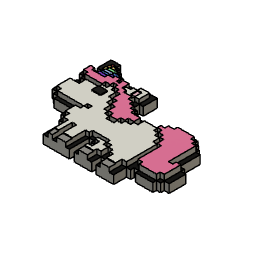
unicorn (Autodesk Fusion 360 design; units mm, degrees)
Autodesk Fusion 360 part; units mm, degrees
note: some values were not read from the file. Chosen so that the rebuilt part matches the saved one: which face or edge a step refers to; which pieces of a blend or face edit are solid.
sketch "Sketch2" plane through (0, 0, 0) normal (0, 0, 1) x (1, 0, 0)
  line L0 (0.8513, 43.4126) -> (0.8513, 31.4048)
  line L1 (0.8513, 31.4048) -> (4, 31.4048)
  line L2 (4, 31.4048) -> (4, 29)
  line L3 (4, 29) -> (7.2062, 29)
  line L4 (7.2062, 29) -> (7.2062, 31.4048)
  line L5 (7.2062, 31.4048) -> (4, 31.4048)
  line L6 (4, 41) -> (4, 31.4048)
  line L7 (4, 41) -> (10.3467, 41)
  line L8 (10.3467, 41) -> (10.3467, 46)
  line L9 (10.3467, 46) -> (19.3248, 46)
  line L10 (19.3248, 46) -> (19.3248, 48.3635)
  line L11 (19.3248, 48.3635) -> (7, 48.3635)
  line L12 (7, 48.3635) -> (7, 46)
  line L13 (7, 46) -> (4, 46)
  line L14 (4, 46) -> (4, 43.4126)
  line L15 (4, 43.4126) -> (0.8513, 43.4126)
  line L16 (1, 58) -> (1, 50.5063)
  line L17 (1, 50.5063) -> (4, 50.5063)
  line L18 (4, 50.5063) -> (4, 55.5959)
  line L19 (4, 55.5959) -> (7, 55.5959)
  line L20 (7, 55.5959) -> (7, 53.5)
  line L21 (7, 53.5) -> (10, 53.5)
  line L22 (10, 53.5) -> (10, 60.5)
  line L23 (10, 60.5) -> (7.5, 60.5)
  line L24 (7.5, 60.5) -> (7.5, 58)
  line L25 (7.5, 58) -> (1, 58)
  line L26 (4, 50.5063) -> (4, 48.3635)
  line L27 (4, 48.3635) -> (7, 48.3635)
  line L28 (7, 50.5063) -> (4, 50.5063)
  line L29 (7, 50.5063) -> (7, 48.3635)
  line L30 (7.5, 60.5) -> (7.5, 67.5)
  line L31 (7.5, 67.5) -> (10.5, 67.5)
  line L32 (10.5, 67.5) -> (10.5, 70.311)
  line L33 (10.5, 70.311) -> (3.9179, 70.311)
  line L34 (3.9179, 70.311) -> (3.9179, 60.5)
  line L35 (3.9179, 60.5) -> (7.5, 60.5)
  line L36 (10.5, 67.5) -> (10.5, 65.3174)
  line L37 (10.5, 65.3174) -> (13, 65.3174)
  line L38 (13, 65.3174) -> (13, 67.5)
  line L39 (13, 67.5) -> (10.5, 67.5)
  line L40 (13, 65.3174) -> (13, 63)
  line L41 (13, 63) -> (16, 63)
  line L42 (16, 63) -> (16, 65.3174)
  line L43 (16, 65.3174) -> (13, 65.3174)
  line L44 (16, 63) -> (16, 60.5)
  line L45 (16, 60.5) -> (20, 60.5)
  line L46 (20, 60.5) -> (20, 63)
  line L47 (20, 63) -> (16, 63)
  line L48 (7.5, 65.3531) -> (10.5, 65.3174)
  line L49 (7.5, 63) -> (10, 63)
  line L50 (10, 63) -> (10.0277, 65.323)
  line L51 (10, 63) -> (13, 63)
  line L52 (10, 63) -> (10, 60.5)
  line L53 (10, 60.5) -> (16, 60.5)
  line L54 (10, 58) -> (16, 58)
  line L55 (16, 58) -> (16, 60.5)
  line L56 (16, 58) -> (20, 58)
  line L57 (20, 58) -> (20, 60.5)
  line L58 (10, 56) -> (16, 56)
  line L59 (16, 56) -> (16, 58)
  line L60 (16, 56) -> (19.3578, 56)
  line L61 (19.3578, 56) -> (19.3578, 58)
  line L62 (10, 53.5) -> (16, 53.5)
  line L63 (16, 53.5) -> (16, 56)
  line L64 (20, 60.5) -> (35, 60.5)
  line L65 (35, 60.5) -> (35, 58)
  line L66 (35, 58) -> (20, 58)
  line L67 (29, 58) -> (29, 56)
  line L68 (29, 56) -> (32, 56)
  line L69 (32, 56) -> (32, 58)
  line L70 (35, 60.5) -> (35, 63)
  line L71 (35, 63) -> (44, 63)
  line L72 (44, 63) -> (44, 53)
  line L73 (44, 53) -> (41, 53)
  line L74 (41, 53) -> (41, 60.5)
  line L75 (41, 60.5) -> (35, 60.5)
  line L76 (19.3248, 48.3635) -> (22.7328, 48.3635)
  line L77 (22.7328, 48.3635) -> (22.7328, 50.7861)
  line L78 (22.7328, 50.7861) -> (19.3248, 50.7861)
  line L79 (19.3248, 50.7861) -> (19.3248, 48.3635)
  line L80 (22.7328, 50.7861) -> (25.6957, 50.7861)
  line L81 (25.6957, 50.7861) -> (25.6957, 53)
  line L82 (25.6957, 53) -> (22.7328, 53)
  line L83 (22.7328, 53) -> (22.7328, 50.7861)
  line L84 (25.6957, 50.7861) -> (25.6957, 48.5145)
  line L85 (25.6957, 48.5145) -> (29, 48.5145)
  line L86 (29, 48.5145) -> (29, 50.7861)
  line L87 (29, 50.7861) -> (25.6957, 50.7861)
  line L88 (29, 48.5145) -> (29, 43.3457)
  line L89 (29, 43.3457) -> (32, 43.3457)
  line L90 (32, 43.3457) -> (32, 48.5145)
  line L91 (32, 48.5145) -> (29, 48.5145)
  line L92 (29, 56) -> (29, 53)
  line L93 (29, 53) -> (32, 53)
  line L94 (32, 53) -> (32, 51)
  line L95 (32, 51) -> (38, 51)
  line L96 (38, 51) -> (38, 53)
  line L97 (38, 53) -> (41, 53)
  line L98 (41.3977, 53) -> (41.3977, 48.3551)
  line L99 (41.3977, 48.3551) -> (38, 48.3551)
  line L100 (38, 48.3551) -> (38, 51)
  line L101 (35, 58) -> (35, 53)
  line L102 (35, 53) -> (38, 53)
  line L103 (35, 58) -> (38, 58)
  line L104 (38, 58) -> (38, 53)
  line L105 (19.3248, 46) -> (19.3248, 41)
  line L106 (19.3248, 41) -> (25.5972, 41)
  line L107 (25.5972, 41) -> (25.5972, 46)
  line L108 (25.5972, 46) -> (19.3248, 46)
  line L109 (32, 43.3457) -> (32, 39)
  line L110 (32, 39) -> (35, 39)
  line L111 (35, 39) -> (35, 43.3457)
  line L112 (35, 43.3457) -> (32, 43.3457)
  line L113 (35, 39) -> (35, 34)
  line L114 (35, 34) -> (38, 34)
  line L115 (38, 34) -> (38, 39)
  line L116 (38, 39) -> (35, 39)
  line L117 (38, 34) -> (38, 31.5)
  line L118 (38, 31.5) -> (41.5, 31.5)
  line L119 (41.5, 31.5) -> (41.5, 34)
  line L120 (41.5, 34) -> (38, 34)
  line L121 (23, 57) -> (23, 55)
  line L122 (23, 55) -> (25, 55)
  line L123 (25, 55) -> (25, 57)
  line L124 (25, 57) -> (23, 57)
  line L125 (41.5, 31.5) -> (41.5, 29)
  line L126 (41.5, 29) -> (47, 29)
  line L127 (47, 29) -> (47, 31.5)
  line L128 (47, 31.5) -> (41.5, 31.5)
  line L129 (47, 31.5) -> (50, 31.5)
  line L130 (50, 31.5) -> (50, 34)
  line L131 (50, 34) -> (47, 34)
  line L132 (47, 34) -> (47, 31.5)
  line L133 (50, 34) -> (54, 34)
  line L134 (54, 34) -> (54, 36.3995)
  line L135 (50, 34) -> (50, 36.3995)
  line L136 (50, 36.3995) -> (54, 36.3995)
  line L137 (41.3977, 48.3551) -> (41.3977, 46)
  line L138 (41.3977, 46) -> (44.4347, 46)
  line L139 (44.4347, 46) -> (44.4347, 48.3551)
  line L140 (44.4347, 48.3551) -> (41.3977, 48.3551)
  line L141 (44.4347, 46) -> (44.4347, 43.5056)
  line L142 (44.4347, 43.5056) -> (47.3315, 43.5056)
  line L143 (47.3315, 43.5056) -> (47.3315, 46)
  line L144 (47.3315, 46) -> (44.4347, 46)
  line L145 (47.3315, 43.5056) -> (47.3315, 41)
  line L146 (47.3315, 41) -> (54, 41)
  line L147 (54, 41) -> (54, 36.3995)
  line L148 (54, 36.3995) -> (56.7414, 36.3995)
  line L149 (56.7414, 36.3995) -> (56.7414, 41.0689)
  line L150 (47.3315, 43.5056) -> (66, 43.5056)
  line L151 (66, 43.5056) -> (66, 46)
  line L152 (66, 46) -> (69, 46)
  line L153 (69, 46) -> (69, 43.5056)
  line L154 (69, 43.5056) -> (66, 43.5056)
  line L155 (56.7414, 41.0689) -> (66, 41.0689)
  line L156 (66, 41.0689) -> (66, 43.5056)
  line L157 (66, 41.0689) -> (66, 38.5034)
  line L158 (66, 38.5034) -> (69.1958, 38.5034)
  line L159 (69.1958, 38.5034) -> (69.1958, 41)
  line L160 (69.1958, 41) -> (66, 41.0689)
  line L161 (69.1958, 38.5034) -> (69.1958, 36)
  line L162 (69.1958, 36) -> (72.6786, 36)
  line L163 (72.6786, 36) -> (72.6786, 38.5034)
  line L164 (72.6786, 38.5034) -> (69.1958, 38.5034)
  line L165 (72.6786, 36) -> (72.6786, 31.3152)
  line L166 (72.6786, 31.3152) -> (75.6137, 31.3152)
  line L167 (75.6137, 31.3152) -> (75.6137, 36)
  line L168 (75.6137, 36) -> (72.6786, 36)
  line L169 (69, 46) -> (73, 46)
  line L170 (73, 46) -> (73, 48.4442)
  line L171 (73, 48.4442) -> (69, 48.4442)
  line L172 (73, 48.4442) -> (73, 51)
  line L173 (73, 51) -> (84.9612, 51)
  line L174 (84.9612, 51) -> (84.9612, 48.4442)
  line L175 (84.9612, 48.4442) -> (73, 48.4442)
  line L176 (84.9612, 48.4442) -> (84.9612, 46)
  line L177 (84.9612, 46) -> (88, 46)
  line L178 (88, 46) -> (88, 48.4442)
  line L179 (88, 48.4442) -> (84.9612, 48.4442)
  line L180 (88, 46) -> (88, 43.5414)
  line L181 (88, 43.5414) -> (91, 43.5414)
  line L182 (91, 43.5414) -> (91, 46)
  line L183 (91, 46) -> (88, 46)
  line L184 (91, 43.5414) -> (91, 24)
  line L185 (91, 24) -> (94, 24)
  line L186 (94, 24) -> (94, 26.4371)
  line L187 (94, 26.4371) -> (97.3699, 26.4371)
  line L188 (97.3699, 26.4371) -> (97.3699, 29)
  line L189 (97.3699, 29) -> (94, 29)
  line L190 (94, 29) -> (94, 43.5414)
  line L191 (94, 43.5414) -> (91, 43.5414)
  line L192 (97.3699, 26.4371) -> (100.8513, 26.4371)
  line L193 (100.8513, 26.4371) -> (100.8513, 14.6247)
  line L194 (100.8513, 14.6247) -> (97.3699, 14.6247)
  line L195 (97.3699, 14.6247) -> (97.3699, 26.4371)
  line L196 (97.3699, 14.6247) -> (94.4082, 14.6247)
  line L197 (94.4082, 14.6247) -> (94.4082, 12)
  line L198 (94.4082, 12) -> (97.3699, 12)
  line L199 (97.3699, 12) -> (97.3699, 14.6247)
  line L200 (94.4082, 12) -> (94.4082, 9.4824)
  line L201 (94.4082, 9.4824) -> (82, 9.4824)
  line L202 (82, 9.4824) -> (82, 12)
  line L203 (82, 12) -> (94.4082, 12)
  line L204 (75.6137, 31.3152) -> (75.6137, 9.4824)
  line L205 (75.6137, 9.4824) -> (78.568, 9.4824)
  line L206 (78.568, 9.4824) -> (78.568, 12)
  line L207 (78.568, 12) -> (82, 12)
  line L208 (82, 14.6135) -> (78.568, 14.6135)
  line L209 (78.568, 14.6135) -> (78.568, 31.3152)
  line L210 (78.568, 31.3152) -> (75.6137, 31.3152)
  line L211 (7.2062, 29) -> (7.2062, 26.2697)
  line L212 (7.2062, 26.2697) -> (19.5, 26.2697)
  line L213 (19.5, 26.2697) -> (19.5, 19)
  line L214 (19.5, 19) -> (22.5, 19)
  line L215 (22.5, 19) -> (22.5, 26.2697)
  line L216 (22.5, 26.2697) -> (26, 26.2697)
  line L217 (26, 26.2697) -> (26, 28.7494)
  line L218 (26, 28.7494) -> (29, 28.7494)
  line L219 (29, 28.7494) -> (29, 31.4907)
  line L220 (29, 31.4907) -> (26, 31.4907)
  line L221 (26, 31.4907) -> (26, 28.7494)
  line L222 (7.2062, 28.7494) -> (26, 28.7494)
  line L223 (22.5, 19) -> (22.5, 14.5)
  line L224 (22.5, 14.5) -> (25.5, 14.5)
  line L225 (25.5, 14.5) -> (25.5, 19)
  line L226 (25.5, 19) -> (22.5, 19)
  line L227 (25.5, 14.5) -> (25.5, 0.311)
  line L228 (25.5, 0.311) -> (29, 0.311)
  line L229 (29, 0.311) -> (29, 14.5)
  line L230 (29, 14.5) -> (25.5, 14.5)
  line L231 (29, 5) -> (32, 5)
  line L232 (32, 5) -> (32, 14.5)
  line L233 (32, 14.5) -> (35, 14.5)
  line L234 (35, 14.5) -> (35, 0.311)
  line L235 (35, 0.311) -> (32, 0.311)
  line L236 (32, 0.311) -> (32, 5)
  line L237 (29, 0.311) -> (32, 0.311)
  line L238 (35, 5) -> (41.5, 5)
  line L239 (41.5, 5) -> (41.5, 0.311)
  line L240 (41.5, 0.311) -> (35, 0.311)
  line L241 (41.5, 5) -> (41.5, 14.4758)
  line L242 (41.5, 14.4758) -> (44.1269, 14.4758)
  line L243 (44.1269, 14.4758) -> (44.1269, 0.311)
  line L244 (44.1269, 0.311) -> (41.5, 0.311)
  line L245 (44.1269, 14.4758) -> (44.1269, 16.7379)
  line L246 (44.1269, 16.7379) -> (56.6416, 16.7379)
  line L247 (56.6416, 16.7379) -> (56.6416, 14.5)
  line L248 (56.6416, 14.5) -> (50.3842, 14.5)
  line L249 (50.3842, 14.5) -> (50.3842, 12.3022)
  line L250 (50.3842, 12.3022) -> (47.537, 12.3022)
  line L251 (47.537, 12.3022) -> (47.537, 14.5)
  line L252 (47.537, 14.5) -> (44.1269, 14.4758)
  line L253 (50.3842, 12.3022) -> (50.3842, 7)
  line L254 (50.3842, 7) -> (53.5129, 7)
  line L255 (53.5129, 7) -> (53.5129, 12.3022)
  line L256 (53.5129, 12.3022) -> (50.3842, 12.3022)
  line L257 (50.3842, 7) -> (47.5323, 7)
  line L258 (47.5323, 7) -> (47.5323, 0.311)
  line L259 (47.5323, 0.311) -> (50.3842, 0.311)
  line L260 (50.3842, 0.311) -> (50.3842, 7)
  line L261 (50.3842, 4.7934) -> (57, 4.7934)
  line L262 (57, 4.7934) -> (57, 0.311)
  line L263 (57, 0.311) -> (50.3842, 0.311)
  line L264 (57, 4.7934) -> (57, 7)
  line L265 (57, 7) -> (60, 7)
  line L266 (60, 7) -> (60, 0.311)
  line L267 (60, 0.311) -> (57, 0.311)
  line L268 (56.6416, 14.5) -> (56.6416, 12)
  line L269 (56.6416, 12) -> (60, 12)
  line L270 (60, 12) -> (60, 14.5)
  line L271 (60, 14.5) -> (56.6416, 14.5)
  line L272 (63.1059, 0.311) -> (66, 0.311)
  line L273 (66, 0.311) -> (66, 9.5985)
  line L274 (66, 9.5985) -> (63.3178, 9.5985)
  line L275 (63.3178, 9.5985) -> (63.3178, 12)
  line L276 (63.3178, 12) -> (60, 12)
  line L277 (66, 4.9547) -> (72.435, 4.9547)
  line L278 (72.435, 4.9547) -> (72.435, 0.311)
  line L279 (72.435, 0.311) -> (66, 0.311)
  line L280 (72.435, 4.9547) -> (72.435, 9.485)
  line L281 (72.435, 9.485) -> (75.6137, 9.4824)
  line L282 (75.6137, 0.311) -> (72.435, 0.311)
  line L283 (75.6137, 0.311) -> (75.6137, 9.4824)
  line L284 (60, 7) -> (63.1059, 7)
  line L285 (63.1059, 7) -> (63.1059, 0.311)
  line L286 (60, 7) -> (60, 12)
  line L287 (82, 14.6135) -> (82, 12)
  line L288 (69, 48.4442) -> (69, 46)
  dimension "d57" = 70
  dimension "d60" = 100
  constraint vertical L0
  constraint perpendicular L0 L1
  constraint perpendicular L1 L2
  constraint perpendicular L2 L3
  constraint perpendicular L1 L4
  constraint perpendicular L4 L5
  constraint perpendicular L1 L6
  constraint perpendicular L6 L7
  constraint perpendicular L7 L8
  constraint perpendicular L8 L9
  constraint perpendicular L9 L10
  constraint perpendicular L10 L11
  constraint perpendicular L11 L12
  constraint perpendicular L12 L13
  constraint perpendicular L11 L14
  constraint perpendicular L0 L15
  constraint vertical L16
  constraint perpendicular L16 L17
  constraint perpendicular L17 L18
  constraint perpendicular L18 L19
  constraint perpendicular L17 L20
  constraint perpendicular L18 L21
  constraint perpendicular L21 L22
  constraint perpendicular L22 L23
  constraint perpendicular L21 L24
  constraint perpendicular L22 L25
  constraint perpendicular L17 L26
  constraint perpendicular L11 L29
  constraint perpendicular L26 L27
  constraint perpendicular L28 L29
  constraint perpendicular L23 L30
  constraint perpendicular L30 L31
  constraint perpendicular L23 L32
  constraint perpendicular L30 L33
  constraint perpendicular L30 L35
  constraint perpendicular L34 L35
  constraint perpendicular L31 L36
  constraint perpendicular L36 L37
  constraint perpendicular L37 L38
  constraint perpendicular L36 L39
  constraint perpendicular L37 L40
  constraint perpendicular L40 L41
  constraint perpendicular L41 L42
  constraint perpendicular L40 L43
  constraint perpendicular L41 L44
  constraint perpendicular L42 L45
  constraint perpendicular L45 L46
  constraint perpendicular L42 L47
  constraint coincident L30 L48.start
  constraint coincident L30 L49.start
  constraint perpendicular L30 L49
  constraint coincident L48 L50.end
  constraint perpendicular L48 L50
  constraint parallel L49 L51
  constraint perpendicular L23 L52
  constraint perpendicular L52 L53
  constraint coincident L22 L54.start
  constraint perpendicular L22 L54
  constraint perpendicular L53 L55
  constraint perpendicular L55 L56
  constraint perpendicular L45 L57
  constraint coincident L22 L58.start
  constraint perpendicular L22 L58
  constraint perpendicular L56 L59
  constraint perpendicular L59 L60
  constraint perpendicular L60 L61
  constraint perpendicular L22 L62
  constraint perpendicular L58 L63
  constraint perpendicular L46 L64
  constraint perpendicular L45 L65
  constraint perpendicular L57 L66
  constraint coincident L66 L67.start
  constraint perpendicular L66 L67
  constraint perpendicular L57 L68
  constraint coincident L66 L69.end
  constraint perpendicular L66 L69
  constraint perpendicular L64 L70
  constraint perpendicular L65 L71
  constraint perpendicular L71 L72
  constraint perpendicular L72 L73
  constraint perpendicular L73 L74
  constraint perpendicular L70 L75
  constraint perpendicular L10 L76
  constraint perpendicular L11 L77
  constraint perpendicular L10 L78
  constraint perpendicular L11 L79
  constraint perpendicular L79 L80
  constraint perpendicular L80 L81
  constraint perpendicular L79 L82
  constraint perpendicular L78 L83
  constraint perpendicular L80 L84
  constraint perpendicular L81 L85
  constraint perpendicular L85 L86
  constraint perpendicular L81 L87
  constraint perpendicular L85 L88
  constraint perpendicular L86 L89
  constraint perpendicular L85 L90
  constraint perpendicular L88 L91
  constraint perpendicular L78 L92
  constraint perpendicular L92 L93
  constraint perpendicular L93 L94
  constraint perpendicular L94 L95
  constraint perpendicular L95 L96
  constraint perpendicular L96 L97
  constraint coincident L73 L98.start
  constraint perpendicular L73 L98
  constraint perpendicular L98 L99
  constraint perpendicular L95 L100
  constraint perpendicular L95 L101
  constraint perpendicular L96 L102
  constraint perpendicular L101 L103
  constraint perpendicular L97 L104
  constraint perpendicular L9 L105
  constraint perpendicular L105 L106
  constraint perpendicular L106 L107
  constraint perpendicular L10 L108
  constraint perpendicular L89 L109
  constraint perpendicular L109 L110
  constraint perpendicular L89 L111
  constraint perpendicular L109 L112
  constraint perpendicular L110 L113
  constraint perpendicular L111 L114
  constraint perpendicular L114 L115
  constraint perpendicular L113 L116
  constraint perpendicular L114 L117
  constraint perpendicular L115 L118
  constraint perpendicular L118 L119
  constraint perpendicular L117 L120
  constraint perpendicular L11 L121
  constraint perpendicular L121 L122
  constraint perpendicular L122 L123
  constraint perpendicular L121 L124
  constraint perpendicular L118 L125
  constraint perpendicular L125 L126
  constraint perpendicular L118 L127
  constraint perpendicular L125 L128
  constraint perpendicular L127 L129
  constraint perpendicular L128 L130
  constraint perpendicular L130 L131
  constraint perpendicular L128 L132
  constraint perpendicular L130 L133
  constraint perpendicular L131 L134
  constraint perpendicular L131 L135
  constraint perpendicular L99 L137
  constraint perpendicular L137 L138
  constraint perpendicular L138 L139
  constraint perpendicular L137 L140
  constraint perpendicular L138 L141
  constraint perpendicular L141 L142
  constraint perpendicular L142 L143
  constraint perpendicular L139 L144
  constraint perpendicular L144 L145
  constraint perpendicular L145 L146
  constraint parallel L134 L147
  constraint perpendicular L148 L149
  constraint perpendicular L147 L148
  constraint perpendicular L134 L136
  constraint perpendicular L143 L150
  constraint perpendicular L150 L151
  constraint perpendicular L151 L152
  constraint perpendicular L152 L153
  constraint perpendicular L151 L154
  constraint perpendicular L149 L155
  constraint perpendicular L150 L156
  constraint perpendicular L155 L157
  constraint perpendicular L157 L158
  constraint perpendicular L158 L159
  constraint perpendicular L158 L161
  constraint perpendicular L159 L162
  constraint perpendicular L158 L163
  constraint perpendicular L161 L164
  constraint perpendicular L162 L165
  constraint perpendicular L165 L166
  constraint perpendicular L166 L167
  constraint perpendicular L167 L168
  constraint perpendicular L153 L169
  constraint perpendicular L169 L170
  constraint perpendicular L153 L171
  constraint perpendicular L171 L172
  constraint perpendicular L170 L173
  constraint perpendicular L171 L174
  constraint perpendicular L172 L175
  constraint perpendicular L175 L176
  constraint perpendicular L176 L177
  constraint perpendicular L177 L178
  constraint perpendicular L174 L179
  constraint perpendicular L177 L180
  constraint perpendicular L180 L181
  constraint perpendicular L177 L182
  constraint perpendicular L180 L183
  constraint perpendicular L181 L184
  constraint perpendicular L184 L185
  constraint perpendicular L185 L186
  constraint perpendicular L186 L187
  constraint perpendicular L187 L188
  constraint perpendicular L188 L189
  constraint perpendicular L189 L190
  constraint perpendicular L190 L191
  constraint perpendicular L188 L192
  constraint perpendicular L192 L193
  constraint perpendicular L188 L194
  constraint perpendicular L192 L195
  constraint perpendicular L195 L196
  constraint perpendicular L194 L197
  constraint perpendicular L197 L198
  constraint perpendicular L194 L199
  constraint perpendicular L198 L200
  constraint perpendicular L200 L201
  constraint perpendicular L198 L202
  constraint perpendicular L200 L203
  constraint perpendicular L166 L204
  constraint perpendicular L204 L205
  constraint perpendicular L166 L206
  constraint perpendicular L202 L207
  constraint perpendicular L202 L208
  constraint perpendicular L208 L209
  constraint perpendicular L209 L210
  constraint perpendicular L3 L211
  constraint perpendicular L4 L212
  constraint perpendicular L212 L213
  constraint perpendicular L213 L214
  constraint perpendicular L214 L215
  constraint perpendicular L215 L216
  constraint perpendicular L214 L217
  constraint perpendicular L217 L218
  constraint perpendicular L214 L219
  constraint perpendicular L217 L220
  constraint coincident L211 L222.start
  constraint perpendicular L211 L222
  constraint perpendicular L220 L221
  constraint perpendicular L214 L223
  constraint perpendicular L215 L224
  constraint perpendicular L214 L225
  constraint perpendicular L223 L226
  constraint perpendicular L224 L227
  constraint perpendicular L225 L228
  constraint perpendicular L228 L229
  constraint perpendicular L227 L230
  constraint coincident L229 L231.start
  constraint perpendicular L229 L231
  constraint perpendicular L224 L232
  constraint perpendicular L229 L233
  constraint perpendicular L224 L234
  constraint perpendicular L229 L235
  constraint perpendicular L231 L236
  constraint perpendicular L236 L237
  constraint coincident L234 L238.start
  constraint perpendicular L234 L238
  constraint perpendicular L238 L239
  constraint perpendicular L234 L240
  constraint perpendicular L238 L241
  constraint perpendicular L241 L242
  constraint perpendicular L239 L244
  constraint perpendicular L242 L243
  constraint perpendicular L242 L245
  constraint perpendicular L243 L246
  constraint perpendicular L246 L247
  constraint perpendicular L247 L248
  constraint perpendicular L246 L249
  constraint perpendicular L249 L250
  constraint perpendicular L250 L251
  constraint perpendicular L250 L253
  constraint perpendicular L249 L254
  constraint perpendicular L250 L255
  constraint perpendicular L253 L256
  constraint perpendicular L253 L257
  constraint perpendicular L254 L258
  constraint perpendicular L258 L259
  constraint perpendicular L257 L260
  constraint perpendicular L253 L261
  constraint perpendicular L257 L262
  constraint perpendicular L260 L263
  constraint perpendicular L261 L264
  constraint perpendicular L262 L265
  constraint perpendicular L265 L266
  constraint perpendicular L262 L267
  constraint perpendicular L248 L268
  constraint perpendicular L247 L269
  constraint perpendicular L248 L270
  constraint perpendicular L247 L271
  constraint perpendicular L270 L272
  constraint perpendicular L269 L273
  constraint perpendicular L270 L274
  constraint perpendicular L269 L275
  constraint perpendicular L270 L276
  constraint midpoint L273 L277.start
  constraint perpendicular L273 L277
  constraint perpendicular L274 L278
  constraint perpendicular L273 L279
  constraint perpendicular L277 L280
  constraint perpendicular L205 L283
  constraint perpendicular L282 L283
  constraint perpendicular L266 L284
  constraint perpendicular L276 L286
  constraint perpendicular L272 L285
  constraint perpendicular L207 L287
  constraint perpendicular L152 L288
  measures "d57" distance of L33 L240
  measures "d60" distance of L0 L193
extrude "Extrude1" add sketch "Sketch2" along normal blind 10 contours L11 L18 L19 L20 L21 L28 L29 L56 L60 L61 L62 L63 L66 L67 L78 L79 L81 L82 L83 L86 L87 L90 L91 L92 L93 L94 L95 L99 L100 L111 L112 L115 L116 L119 L120 L128 L131 L132 L135 L136 L137 L138 L141 L142 L145 L146 L147
extrude "Extrude2" add sketch "Sketch2" along normal blind 9.5 contours L22 L58 L62 L63 | L56 L59 L60 L61
extrude "Extrude3" add sketch "Sketch2" along normal blind 9.2 contours L22 L54 L58 L59 | L45 L55 L56 L57
extrude "Extrude4" add sketch "Sketch2" along normal blind 9 contours L22 L53 L54 L55
extrude "Extrude5" add sketch "Sketch2" along normal blind 8.7 contours L41 L44 L51 L52 L53
delete_face "DeleteFace1" 1 faces at (12, 62.1667, 8.7)
delete_face "DeleteFace2" 2 faces at (12, 60.5, 3) (12, 59.6667, 9)
delete_face "DeleteFace3" 2 faces at (12, 57.3333, 9.2) (12, 58, 3.0667)
delete_face "DeleteFace4" 3 faces at (12, 55.1667, 9.5) (10, 55.1667, 3.1667) (12, 56, 3.1667)
delete_face "DeleteFace5" 5 faces at (16, 57.3333, 3.0667) (17.3333, 60.5, 6.1333) (17.3333, 59.6667, 9.2) (17.1193, 57.3333, 9.5) (20, 58.8333, 3.0667)
extrude "Extrude6" add sketch "Sketch2" along normal blind 9.5 contours L22 L58 L62 L63 | L56 L59 L60 L61
extrude "Extrude7" add sketch "Sketch2" along normal blind 9 contours L22 L54 L58 L59 | L45 L55 L56 L57
extrude "Extrude8" add sketch "Sketch2" along normal blind 8.5 contours L22 L53 L54 L55
extrude "Extrude9" add sketch "Sketch2" along normal blind 8 contours L41 L44 L51 L52 L53
extrude "Extrude10" add sketch "Sketch2" along normal blind 7.5 contours L23 L30 L49 L52 | L37 L40 L48 L50 L51
extrude "Extrude11" add sketch "Sketch2" along normal blind 7 contours L30 L48 L49 L50
extrude "Extrude12" add sketch "Sketch2" along normal blind 6.5 contours L30 L31 L36 L48
extrude "Extrude13" add sketch "Sketch2" along normal blind 9 contours L66 L68 L69 L92 L93 L94 L95 L96 L101 L102
extrude "Extrude14" add sketch "Sketch2" along normal blind 8.5 contours L101 L102 L103 L104
extrude "Extrude15" add sketch "Sketch2" along normal blind 9 contours L65 L74 L75 L97 L103 L104
extrude "Extrude16" add sketch "Sketch2" along normal blind 6 contours L0 L1 L6 L7 L8 L9 L10 L11 L12 L13 L14 L15 | L26 L27 L28 L29 | L76 L77 L78 L79 | L16 L17 L18 L19 L20 L21 L22 L23 L24 L25 | L80 L81 L82 L83 | L84 L85 L86 L87 | L88 L89 L90 L91 | L30 L31 L32 L33 L34 L35 | L109 L110 L111 L112 | L44 L45 L46 L47 | L40 L41 L42 L43 | L57 L64 L65 L66 | L113 L114 L115 L116 | L36 L37 L38 L39 | L70 L71 L72 L73 L74 L75 | L66 L67 L68 L69 | L117 L118 L119 L120 | L73 L96 L97 L98 L99 L100 | L125 L126 L127 L128 | L137 L138 L139 L140 | L129 L130 L131 L132 | L141 L142 L143 L144 | L133 L134 L135 L136 | L145 L146 L147 L148 L149 L150 L155 L156
extrude "Extrude17" add sketch "Sketch2" along normal blind 9.5 contours L4 L5 L6 L7 L8 L9 L10 L76 L77 L80 L84 L85 L88 L89 L109 L110 L113 L114 L117 L118 L125 L126 L127 L129 L130 L133 L134 L148 L149 L155 L157 L158 L161 L162 L165 L166 L204 L211 L215 L216 L217 L222 L225 L226 L229 L230 L231 L232 L233 L234 L238 L241 L242 L245 L246 L247 L270 L271 L273 L274 L275 L276 L277 L280 L281
extrude "Extrude18" add sketch "Sketch2" along normal blind 10 contours L105 L106 L107 L108
extrude "Extrude19" add sketch "Sketch2" along normal blind 6 contours L157 L158 L159 L160 | L161 L162 L163 L164 | L165 L166 L167 L168 | L204 L205 L206 L207 L208 L209 L210 L287
extrude "Extrude20" add sketch "Sketch2" along normal blind 10 contours L153 L154 L156 L159 L160 L163 L164 L167 L168 L169 L170 L175 L176 L177 L180 L181 L184 L185 L186 L187 L195 L196 L197 L203 L208 L209 L210 L287
extrude "Extrude21" add sketch "Sketch2" along normal blind 6 contours L151 L152 L153 L154 | L169 L170 L171 L288 | L172 L173 L174 L175 | L176 L177 L178 L179 | L180 L181 L182 L183 | L184 L185 L186 L187 L188 L189 L190 L191 | L200 L201 L202 L203 | L196 L197 L198 L199 | L192 L193 L194 L195
extrude "Extrude22" add sketch "Sketch2" along normal blind 6 contours L2 L3 L4 L5 | L218 L219 L220 L221 | L211 L212 L213 L214 L215 L216 L217 L222 | L223 L224 L225 L226 | L227 L228 L229 L230 | L232 L233 L234 L235 L236 | L239 L241 L242 L243 L244 | L245 L246 L247 L248 L249 L250 L251 L252 | L268 L269 L270 L271 | L272 L273 L274 L275 L276 L284 L285 L286 | L278 L280 L281 L282 L283
extrude "Extrude24" add sketch "Sketch2" along normal blind 9.5 contours L248 L249 L254 L255 L256 L260 L261 L264 L265 L268 L269 L286
extrude "Extrude25" add sketch "Sketch2" along normal blind 6 contours L253 L254 L255 L256 | L257 L258 L259 L260 | L262 L264 L265 L266 L267
extrude "Extrude26" add sketch "Sketch2" along normal blind 9 contours L229 L231 L236 L237 | L234 L238 L239 L240 | L260 L261 L262 L263 | L273 L277 L278 L279
